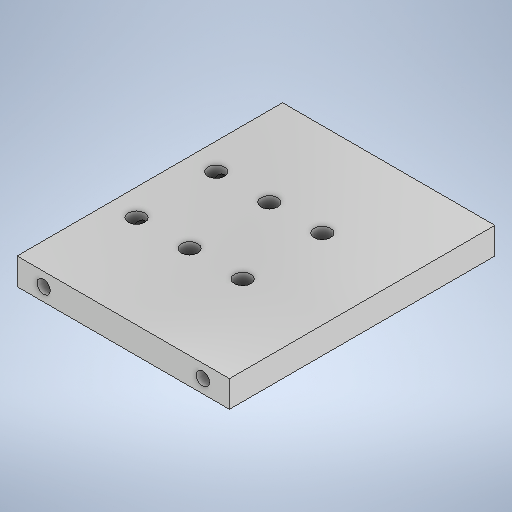
# Autodesk Inventor part: hand2_11
Saved by Autodesk Inventor 2025.1 (Build 291241000, 241)
## iProperties
Created: 2025-02-03
Part Number: hand2_11
Material: アルミニウム 6061-AHC
Document SubType Name: Modeling
Designer: ryogo
Density: 2.7 g/cm^3
Appearance: アルミニウム - ダーク
Author: ryogo
Autodesk Inventor part; units mm, degrees
ref_plane "YZ Plane" through (0, 0, 0) normal (1, 0, 0) x (0, 1, 0)
ref_plane "XZ Plane" through (0, 0, 0) normal (0, 1, 0) x (-1, 0, 0)
ref_plane "XY Plane" through (0, 0, 0) normal (0, 0, 1) x (1, 0, 0)
sketch "スケッチ1" plane through (0, 0, 0) normal (0, 1, 0) x (-1, 0, 0)
  line L0 (0, 0) -> (40, 0)
  line L1 (40, 0) -> (40, -50)
  line L2 (40, -50) -> (0, -50)
  line L3 (0, -50) -> (0, 0)
  line L4 (35, -50) -> (35, 0)
  line L5 (30, -50) -> (30, 0)
  line L6 (25, -50) -> (25, 0)
  line L7 (20, -50) -> (20, 0)
  line L8 (15, -50) -> (15, 0)
  line L9 (10, -50) -> (10, 0)
  line L10 (5, -50) -> (5, 0)
  dimension "d0" = 40
  dimension "d1" = 50
  dimension "d2" = 5
  dimension "d6" = 5
  constraints: 22 end point, 2 horizontal, 2 parallel, 2 perpendicular, 2 point on line, 18 other
  measures "d0" distance of L1.end L2.end
  measures "d1" distance of L0.end L1.end
  measures "d2" distance between parallel lines of L1 L4
  measures "d6" distance of L4.start L5.start
extrude "押し出し1" add sketch "スケッチ1" along normal blind 5
sketch "スケッチ4" plane through (0, 0, 0) normal (0, -1, 0) x (1, 0, 0)
  line L0 (-40, -50) -> (-40, 0) projected
  line L1 (-40, -17.5) -> (0, -17.5)
  line L2 (0, 0) -> (0, -50) projected
  line L3 (0, -32.5) -> (-35, -32.5)
  line L4 (-40, 0) -> (0, 0) projected
  line L5 (0, -50) -> (-40, -50) projected
  line L6 (-25, -50) -> (-25, 0) projected
  line L7 (-20, -50) -> (-20, 0) projected
  line L8 (-15, -50) -> (-15, 0) projected
  line L9 (-40, -25) -> (0, -25)
  point P0 (-25, -17.5)
  point P1 (-15, -17.5)
  point P2 (-15, -32.5)
  point P3 (-25, -32.5)
  dimension "d49" = 15
  dimension "d50" = 15
  constraints: 11 point on line, 6 end point, 2 horizontal, 2 midpoint, 2 parallel
  measures "d49" diameter of L9 L1
  measures "d50" diameter of L9 L3
hole "穴3" at (-15, 0, -17.5) at (-15, 0, -32.5) at (-25, 0, -17.5) at (-25, 0, -32.5) direction (0, 1, 0) diameter 3.1 end through all
sketch "スケッチ5" plane through (0, 0, -50) normal (0, 0, -1) x (-1, 0, 0)
  line L0 (40, 0) -> (40, 5) projected
  line L1 (40, 2.5) -> (0, 2.5)
  line L2 (0, 0) -> (0, 5) projected
  point P0 (35, 0)
  point P1 (35, 0)
  point P2 (35, 0)
  point P3 (5, 0)
  point P4 (5, 0)
  point P5 (5, 0)
  point P6 (35, 2.5)
  point P7 (5, 2.5)
  constraints: 2 end point, 2 midpoint, 2 point on line
hole "穴4" at (-35, 2.5, -50) at (-5, 2.5, -50) direction (0, 0, 1) diameter 2.5 end through all
sketch "スケッチ6" plane through (0, 5, 0) normal (0, 1, 0) x (1, 0, 0)
  line L0 (-40, 0) -> (0, 0) projected
  line L1 (-35, 0) -> (-35, 50)
  line L2 (-6.25, 0) -> (-6.25, 50) projected
  circle A0 centre (-15, 32.5) radius 1.55 projected
  circle A1 centre (-25, 32.5) radius 1.55 projected
  point P0 (-35, 32.5)
  point P1 (-35, 17.5)
  dimension "d52" = 15
  dimension "d60" = 10
  constraints: 3 point on line, 2 end point, 1 parallel
  measures "d52" distance of point (-35, 17.5) point (-35, 32.5)
  measures "d60" distance from line of L1 A1.centre
hole "穴5" at (-35, 5, -32.5) at (-35, 5, -17.5) direction (0, -1, 0) diameter 3.1 end through all
